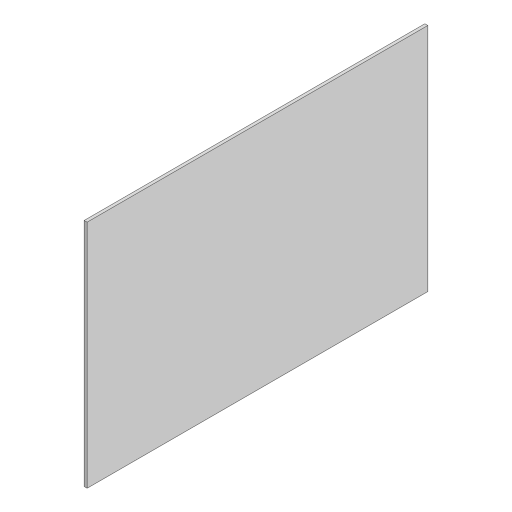
# Autodesk Inventor part: CUT PART J
Saved by Autodesk Inventor 2023.1 (Build 271208000, 208)
## iProperties
Created: 2022-11-02
Part Number: CUT PART J
Material: Generic
Document SubType Name: Modeling
Designer: GUT
Density: 1 g/cm^3
Appearance: Default
Author: GUT
Autodesk Inventor part; units mm, degrees
ref_plane "YZ Plane" through (0, 0, 0) normal (1, 0, 0) x (0, 1, 0)
ref_plane "XZ Plane" through (0, 0, 0) normal (0, 1, 0) x (-1, 0, 0)
ref_plane "XY Plane" through (0, 0, 0) normal (0, 0, 1) x (1, 0, 0)
sketch "Sketch1" plane through (0, 0, 0) normal (1, 0, 0) x (0, 1, 0)
  line L0 (-6.2078, 21.6915) -> (457.7922, 21.6915)
  line L1 (457.7922, 21.6915) -> (457.7922, -664.3085)
  line L2 (457.7922, -664.3085) -> (-6.2078, -664.3085)
  line L3 (-6.2078, -664.3085) -> (-6.2078, 21.6915)
  point P0 (0, 0)
  dimension "d0" = 464
  dimension "b" = 686
  constraints: 8 end point, 2 parallel, 1 horizontal, 1 perpendicular
  measures "d0" distance of L1.end L2.end
  measures "b" distance of L0.end L1.end
extrude "Extrusion1" add sketch "Sketch1" along normal blind 6
body "Solid1"
